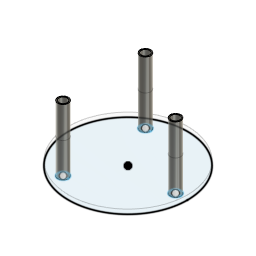
IRLocalization v8 (Autodesk Fusion 360 design; units mm, degrees)
Autodesk Fusion 360 part; units mm, degrees
sketch "Sketch1" plane through (0, 0, 0) normal (0, 0, 1) x (1, 0, 0) in component "Base"
  circle A0 centre (0, 0) radius 40
  circle A1 centre (32, 0) radius 3.5
  circle A2 centre (-16, 27.71) radius 3.5
  circle A3 centre (-16, -27.71) radius 3.5
  circle A4 centre (-16, -27.71) radius 2.5
  circle A5 centre (32, 0) radius 2.5
  circle A6 centre (-16, 27.71) radius 2.5
  dimension "d1" = 80
  dimension "d2" = 7
  dimension "d3" = 7
  dimension "d4" = 7
  dimension "d7" = 5
  dimension "d8" = 5
  dimension "d9" = 5
  constraint coincident A0.centre origin
  constraint concentric A3 A4
  constraint concentric A1 A5
  constraint concentric A2 A6
  measures "d1" diameter of A0
  measures "d2" diameter of A1
  measures "d3" diameter of A2
  measures "d4" diameter of A3
  measures "d7" diameter of A4
  measures "d8" diameter of A5
  measures "d9" diameter of A6
extrude "Extrude1" add sketch "Sketch1" along normal blind 3 contours A0 | A1 | A2 | A3 | A4 | A5 | A6 makes body 1 in component "Base"
extrude "Extrude2" add sketch "Sketch1" along normal blind 23 separate body contours A1 | A2 | A3 | A4 | A5 | A6 makes body 2 at (-12.5044, 27.5355, 15.3333) makes body 3 at (35.4956, -0.1745, 15.3333) makes body 4 at (-12.5044, -27.8845, 15.3333) in component "Base"
extrude "Extrude3" add sketch "Sketch1" along normal blind 30 separate body contours A4 | A5 | A6 makes body 5 at (-13.5124, 27.4611, 20) makes body 6 at (34.4876, -0.2489, 20) makes body 7 at (-13.5124, -27.9589, 20) in component "Base"
copy_body "CutPasteBodies1" bodies 1 2 3 4 5 6 7 removing the originals makes body 8 makes body 9 makes body 10 makes body 11 makes body 12 makes body 13 makes body 14 in component "Base"
sketch "Sketch1 (2)" plane through (0, 0, 0) normal (0, 0, 1) x (1, 0, 0) in component "Top"
  circle A0 centre (0, 0) radius 40
  circle A1 centre (-16, 27.71) radius 2.75
  circle A2 centre (-16, 27.71) radius 3.5
  circle A3 centre (-16, -27.71) radius 2.75
  circle A4 centre (-16, -27.71) radius 3.5
  circle A5 centre (32, 0) radius 2.75
  circle A6 centre (32, 0) radius 3.5
  dimension "d19" = 80
  dimension "d22" = 5.5
  dimension "d23" = 7
  dimension "d24" = 5.5
  dimension "d25" = 7
  dimension "d26" = 5.5
  dimension "d27" = 7
  constraint coincident A0.centre origin
  constraint concentric A1 A2
  constraint concentric A3 A4
  constraint concentric A5 A6
  measures "d19" diameter of A0
  measures "d22" diameter of A1
  measures "d23" diameter of A2
  measures "d24" diameter of A3
  measures "d25" diameter of A4
  measures "d26" diameter of A5
  measures "d27" diameter of A6
extrude "Extrude7" add sketch "Sketch1 (2)" along normal blind 39 separate body contours A1 | A3 | A5 makes body 15 at (-13.2534, 27.5729, 26) makes body 16 at (-13.2534, -27.8471, 26) makes body 17 at (34.7466, -0.1371, 26) in component "Top"
extrude "Extrude8" add sketch "Sketch1 (2)" along normal blind 44 contours A2 | A4 | A6 bodies 15 16 17 in component "Top"
component "Base" placed x (1, 0, 0) y (0, 1, 0) z (0, 0, 1) at (0, 0, 0)
component "Top" placed x (1, 0, 0) y (0, 1, 0) z (0, 0, 1) at (0, 0, 0)
equation "d2 = Outer"
equation "d3 = Outer"
equation "d4 = Outer"
equation "Outer = 7 mm"
equation "Through = 5.0 mm" comment "0.5mm Tolerance"
equation "d7 = Through"
equation "d8 = Through"
equation "d9 = Through"
equation "Base = 3 mm"
equation "Height = 23 mm"
equation "ThroughHeight = 30 mm"
equation "d15 = Height"
equation "d17 = ThroughHeight"
equation "d22 = ThroughIn"
equation "d23 = Outer"
equation "d24 = ThroughIn"
equation "d25 = Outer"
equation "d26 = ThroughIn"
equation "d27 = Outer"
equation "ThroughIn = 5.5 mm" comment "0.5mm Tolerance"
equation "TopHeight = 44 mm" comment "4mm Emitter Height included"
equation "TopThrough = 39 mm" comment "4mm Emitter Height included"
equation "d43 = TopThrough"
equation "d45 = TopHeight"
